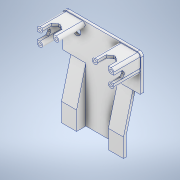
# Autodesk Inventor part: MainHolder
Saved by Autodesk Inventor 2020.2 (Build 242310000, 310)
## iProperties
Created: 2020-01-19
Part Number: MainHolder
Material: Aluminum 6061
Document SubType Name: Modeling
Designer: Paul Lefeuvre
Density: 2.7 g/cm^3
Appearance: Aluminum - Flat
Mass: 1240.34 g
Surface Area: 1399.04 cm^2
Volume: 459.386 cm^3
Author: Paul Lefeuvre
Autodesk Inventor part; units mm, degrees
ref_plane "YZ Plane" through (0, 0, 0) normal (1, 0, 0) x (0, 1, 0)
ref_plane "XZ Plane" through (0, 0, 0) normal (0, 1, 0) x (-1, 0, 0)
ref_plane "XY Plane" through (0, 0, 0) normal (0, 0, 1) x (1, 0, 0)
sketch "Sketch1" plane through (0, 0, 0) normal (0, 0, 1) x (1, 0, 0)
  circle A0 centre (-70.6375, 41.065) radius 20.6375 construction
  line L0 (-45, -24.5725) -> (-45, 76.0179) construction
  line L1 (0, 76.0179) -> (-100.0785, 76.0179)
  line L2 (-109.5785, 66.5179) -> (-109.5785, -22.5725)
  line L3 (-107.5785, -24.5725) -> (0, -24.5725)
  circle A1 centre (-54.5, 66.5179) radius 9.5 construction
  line L4 (-70.6375, 20.4275) -> (-147.8944, 20.4275) construction
  circle A2 centre (-100.0785, 30.9275) radius 10.5 construction
  circle A3 centre (-100.0785, 66.5179) radius 9.5
  circle A4 centre (-100.0785, 66.5179) radius 3 construction
  circle A5 centre (-54.5, 66.5179) radius 3 construction
  circle A6 centre (-100.0785, 30.9275) radius 3 construction
  circle A7 centre (-100.0785, 66.5179) radius 3.6
  circle A8 centre (-54.5, 66.5179) radius 3.6
  circle A9 centre (-100.0785, 30.9275) radius 3.6
  line L5 (0, 0) -> (0, 94.9094) construction
  circle A10 centre (-100.0785, 30.9275) radius 9.5 construction
  circle A11 centre (-100.0785, 66.5179) radius 7.5
  circle A12 centre (-54.5, 66.5179) radius 7.5
  circle A13 centre (-100.0785, 30.9275) radius 7.5
  circle A14 centre (-70.6375, 41.065) radius 10.5 construction
  circle A15 centre (-70.6375, 41.065) radius 11.1
  circle A16 centre (0, -125.7225) radius 21.15 construction
  line L6 (-52.3, -24.5725) -> (-52.3, -178.0225)
  line L7 (-52.3, -178.0225) -> (52.3, -178.0225)
  line L8 (52.3, -178.0225) -> (52.3, -24.5725)
  line L9 (-107.5785, 66.5179) -> (-107.5785, 59.0179)
  line L10 (-107.5785, 59.0179) -> (-100.0785, 59.0179)
  line L11 (-100.0785, 74.0179) -> (-92.5785, 74.0179)
  line L12 (-92.5785, 74.0179) -> (-92.5785, 66.5179)
  line L13 (-107.577, 31.0806) -> (-107.427, 38.4275)
  line L14 (-100.0785, 38.4275) -> (-107.427, 38.4275)
  line L15 (-54.5, 74.0179) -> (-62, 74.0179)
  line L16 (-62, 74.0179) -> (-62, 66.5179)
  circle A17 centre (70.6375, 41.065) radius 20.6375 construction
  line L17 (45, -24.5725) -> (45, 76.0179) construction
  line L18 (0, 76.0179) -> (100.0785, 76.0179)
  line L19 (109.5785, 66.5179) -> (109.5785, -22.5725)
  line L20 (107.5785, -24.5725) -> (0, -24.5725)
  circle A18 centre (54.5, 66.5179) radius 9.5 construction
  circle A19 centre (100.0785, 30.9275) radius 10.5 construction
  circle A20 centre (100.0785, 66.5179) radius 9.5
  circle A21 centre (100.0785, 66.5179) radius 3 construction
  circle A22 centre (54.5, 66.5179) radius 3 construction
  circle A23 centre (100.0785, 30.9275) radius 3 construction
  circle A24 centre (100.0785, 66.5179) radius 3.6
  circle A25 centre (54.5, 66.5179) radius 3.6
  circle A26 centre (100.0785, 30.9275) radius 3.6
  circle A27 centre (100.0785, 30.9275) radius 9.5 construction
  circle A28 centre (100.0785, 66.5179) radius 7.5
  circle A29 centre (54.5, 66.5179) radius 7.5
  circle A30 centre (100.0785, 30.9275) radius 7.5
  circle A31 centre (70.6375, 41.065) radius 10.5 construction
  circle A32 centre (70.6375, 41.065) radius 11.1
  line L21 (107.5785, 66.5179) -> (107.5785, 59.0179)
  line L22 (107.5785, 59.0179) -> (100.0785, 59.0179)
  line L23 (100.0785, 74.0179) -> (92.5785, 74.0179)
  line L24 (92.5785, 74.0179) -> (92.5785, 66.5179)
  line L25 (107.577, 31.0806) -> (107.427, 38.4275)
  line L26 (100.0785, 38.4275) -> (107.427, 38.4275)
  line L27 (54.5, 74.0179) -> (62, 74.0179)
  line L28 (62, 74.0179) -> (62, 66.5179)
  arc A33 (-109.5785, -22.5725) -> (-107.5785, -24.5725) centre (-107.5785, -22.5725) ccw
  arc A34 (107.5785, -24.5725) -> (109.5785, -22.5725) centre (107.5785, -22.5725) ccw
  point P0 (-109.5785, -24.5725)
  point P1 (109.5785, -24.5725)
  point P2 (70.6375, 20.4275)
  point P3 (62, 66.5179)
  dimension "d6" = 21
  dimension "d7" = 41.275
  dimension "d20" = 15
  dimension "d5" = 19
  dimension "d8" = 65.6375
  dimension "d9" = 19
  dimension "d10" = 6
  dimension "d11" = 6
  dimension "d12" = 6
  dimension "d13" = 0.6
  dimension "d14" = 0.6
  dimension "d15" = 0.6
  dimension "d16" = 25.6375
  dimension "d17" = 45
  dimension "d18" = 19
  dimension "d19" = 15
  dimension "d21" = 15
  dimension "d22" = 21
  dimension "d23" = 0.6
  dimension "d24" = 42.3
  dimension "d26" = 101.15
  dimension "d27" = 52.3
  dimension "d28" = 52.3
  dimension "d29" = 52.3
  dimension "d34" = 2
  constraints: 58 end point, 30 symmetric about line, 29 centre point, 20 point on circle, 16 coincident, 13 point on line, 13 tangent, 8 vertical, 6 horizontal, 5 perpendicular, 2 vertical alignment, 1 equal radius, 31 other
  measures "d5" diameter of A1
  measures "d8" distance from line of L3 point (-70.638, 41.065)
  measures "d9" diameter of A3
  measures "d10" diameter of A4
  measures "d11" diameter of A5
  measures "d12" diameter of A6
  measures "d13" radial gap between concentric circles of A4 A7
  measures "d14" radial gap between concentric circles of A5 A8
  measures "d15" radial gap between concentric circles of A6 A9
  measures "d16" distance from line of point (-70.638, 41.065) L0
  measures "d17" distance between parallel lines of L5 L0
  measures "d18" diameter of A10
  measures "d19" diameter of A11
  measures "d21" diameter of A13
  measures "d22" diameter of A14
  measures "d23" radial gap between concentric circles of A14 A15
  measures "d24" diameter of A16
  measures "d26" distance from line of A16.centre L3
  measures "d27" distance from line of L6 A16.centre
  measures "d28" distance from line of L8 A16.centre
  measures "d29" distance from line of A16.centre L7
  measures "d34" radius of A33
extrude "Extrusion1" add sketch "Sketch1" along normal blind 7.5 contours L18 A20 L23 L24 L22 L21 L19 A34 L20 L3 A33 L2 A3 L9 L10 L12 L11 L1 | A3 L11 A11 L9 | A20 L21 A28 L23 | A3 L10 A11 L12 | L24 A28 L22 A20 | L3 L20 L8 L7 L6
extrude "Extrusion2" add sketch "Sketch1" along normal blind 81.5 contours L11 L12 A3 | A3 L12 A11 L11 | L23 A28 L24 A20 | A20 L24 L23 | L9 A11 L10 A3 | A3 L10 L9 | A11 | L21 L22 A20 | A20 L22 A28 L21 | A28 | A12 | A12 L16 L15 | A13 | A13 L13 L14 | A29 | A29 L27 L28 | A30 | A30 L26 L25
sketch "Sketch3" plane through (-52.3, -178.0225, 0) normal (-1, 0, 0) x (0, 0, 1)
  line L0 (0, 0) -> (52.5, 0)
  line L1 (52.5, 0) -> (52.5, 153.45)
  line L2 (52.5, 153.45) -> (0, 153.45)
  line L3 (0, 153.45) -> (0, 0)
  line L4 (26.25, 0) -> (26.25, 52.3)
  line L5 (33.75, 0) -> (33.75, 52.3)
  line L6 (7.5, 153.45) -> (7.5, 0) projected
  line L7 (33.75, 52.3) -> (7.5, 153.45)
  line L8 (0, 0) -> (0, 153.45) projected
  line L9 (26.25, 52.3) -> (0, 153.45)
  point P0 (0, 178.0225)
  point P1 (0, 153.45)
  dimension "d38" = 52.3
  dimension "d39" = 7.5
  dimension "d40" = 18.75
  constraints: 16 end point, 3 parallel, 2 vertical, 1 coincident, 1 horizontal, 1 midpoint, 1 perpendicular, 1 point on line
  measures "d38" distance of L4.start L4.end
  measures "d39" distance between parallel lines of L4 L5
  measures "d40" distance between parallel lines of L6 L4
extrude "Extrusion3" add sketch "Sketch3" along normal blind 35 contours L2 L6 L9 | L4 L9 L6 L7 L5 L0
extrude "Extrusion4" add sketch "Sketch3" against normal blind 7.5 contours L6 L9 L4 L0 | L4 L9 L6 L7 L5 L0
sketch "Sketch4" plane through (-107.5785, 59.0179, 7.5) normal (-1, 0, 0) x (0, 0, 1)
  point P0 (-7.5, -59.0179)
sketch "Sketch6" plane through (-107.5785, 59.0179, 7.5) normal (-1, 0, 0) x (0, 0, 1)
  line L0 (0, 0) -> (74, 0) projected
  line L1 (50, 0) -> (44.7993, -7.4273)
  line L2 (44.7993, -13.1631) -> (50, -20.5904)
  line L3 (0, -20.5904) -> (74, -20.5904) projected
  line L4 (0, 7.5) -> (0, -81.5904) projected
  arc A0 (44.7993, -7.4273) -> (44.7993, -13.1631) centre (48.8951, -10.2952) ccw
  line L5 (50, 0) -> (0, 0)
  line L6 (0, 0) -> (0, -20.5904)
  line L7 (0, -20.5904) -> (50, -20.5904)
  point P0 (-7.5, -59.0179)
  dimension "d51" = 50
  dimension "d52" = 50
  dimension "d54" = 110
  dimension "d55" = 5
  constraints: 10 end point, 2 collinear, 2 point on circle, 2 point on line, 2 tangent, 1 centre point, 1 equal length
  measures "d51" distance from line of L4 L1.start
  measures "d52" distance from line of L4 L2.end
  measures "d54" angle of L1 L2
  measures "d55" radius of A0
extrude "Extrusion5" add sketch "Sketch6" against normal blind 7.5
sketch "Sketch7" plane through (-100.0785, 74.0179, 7.5) normal (0, 1, 0) x (1, 0, 0)
  line L0 (7.5, 0) -> (7.5, -74) projected
  line L1 (7.5, -50) -> (19.9214, -41.3024)
  line L2 (25.6572, -41.3024) -> (38.0785, -50)
  line L3 (38.0785, 0) -> (38.0785, -74) projected
  line L4 (200.1571, 0) -> (0, 0) projected
  arc A0 (25.6572, -41.3024) -> (19.9214, -41.3024) centre (22.7893, -45.3982) ccw
  line L5 (38.0785, -50) -> (38.0785, 0)
  line L6 (38.0785, 0) -> (7.5, 0)
  line L7 (7.5, 0) -> (7.5, -50)
  point P0 (100.0785, 7.5)
  dimension "d58" = 110
  dimension "d59" = 50
  dimension "d60" = 50
  dimension "d61" = 5
  constraints: 10 end point, 2 point on circle, 2 point on line, 2 tangent, 1 centre point, 1 collinear, 1 equal length, 1 perpendicular, 1 vertical
  measures "d58" angle of L2 L1
  measures "d59" distance from line of L4 L2.end
  measures "d60" distance from line of L4 L1.start
  measures "d61" radius of A0
extrude "Extrusion6" add sketch "Sketch7" against normal blind 7.5
ref_plane "Work Plane1" through (0, 0, 0) normal (1, 0, 0) x (0, 1, 0)
mirror "Mirror1" about plane through (0, 0, 0) normal (1, 0, 0) of "Extrusion3", "Extrusion4", "Extrusion6", "Extrusion5"
equation "\"d28\" = d27"
equation "\"d29\" = d27"
equation "\"d51\" = d52"
equation "\"d59\" = d60"
body "Solid1"
